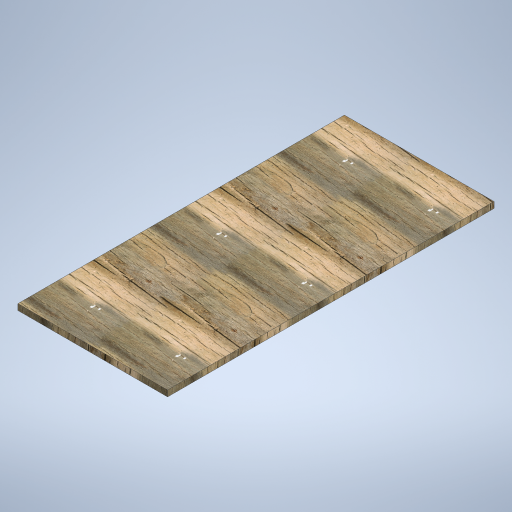
# Autodesk Inventor part: UpperHalfofSides_Ocampo
Saved by Autodesk Inventor 2023 (Build 270158000, 158)
## iProperties
Created: 2025-03-05
Part Number: UpperHalfofSides_Ocampo
Material: Generic
Document SubType Name: Modeling
Designer: FrameUser
Density: 1 g/cm^3
Appearance: Default
Author: FrameUser
Autodesk Inventor part; units mm, degrees
ref_plane "YZ Plane" through (0, 0, 0) normal (1, 0, 0) x (0, 1, 0)
ref_plane "XZ Plane" through (0, 0, 0) normal (0, 1, 0) x (-1, 0, 0)
ref_plane "XY Plane" through (0, 0, 0) normal (0, 0, 1) x (1, 0, 0)
sketch "Sketch1" plane through (0, 0, 0) normal (0, 1, 0) x (-1, 0, 0)
  line L0 (0, 0) -> (-157.1625, 0)
  line L1 (-157.1625, 0) -> (-157.1625, -342.9)
  line L2 (-157.1625, -342.9) -> (0, -342.9)
  line L3 (0, -342.9) -> (0, 0)
  dimension "d0" = 157.1625
  dimension "d1" = 342.9
  constraints: 8 end point, 3 perpendicular, 1 horizontal
  measures "d0" distance of L0.start L0.end
  measures "d1" distance of L0.end L1.end
extrude "Extrusion1" add sketch "Sketch1" along normal blind 6.35
body "Solid1"
